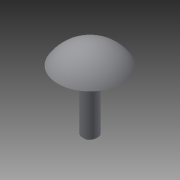
# Autodesk Inventor part: Linkage Peg
Saved by Autodesk Inventor 2015 (Build 190159000, 159)
## iProperties
Created: 2018-03-27
Part Number: Linkage Peg
Material: Generic
Document SubType Name: Modeling
Designer: Administrator
Density: 1 g/cm^3
Appearance: Default
Author: Administrator
Autodesk Inventor part; units mm, degrees
ref_plane "YZ Plane" through (0, 0, 0) normal (1, 0, 0) x (0, 1, 0)
ref_plane "XZ Plane" through (0, 0, 0) normal (0, 1, 0) x (-1, 0, 0)
ref_plane "XY Plane" through (0, 0, 0) normal (0, 0, 1) x (1, 0, 0)
sketch "Sketch1" plane through (0, 0, 0) normal (0, 0, 1) x (1, 0, 0)
  line L0 (0, 0) -> (0, 8.255)
  line L1 (0, 0) -> (0.7938, 0)
  line L2 (0.7938, 0) -> (0.7937, 6.35)
  arc A0 (3.3337, 6.35) -> (0, 8.255) centre (-0.0557, 4.2879) ccw
  line L3 (0.7937, 6.35) -> (3.3337, 6.35)
  dimension "d0" = 3.9675
  dimension "d1" = 6.35
  dimension "d2" = 8.255
  dimension "d3" = 0.7937
  dimension "d4" = 2.54
  constraints: 8 end point, 2 horizontal, 2 point on circle, 1 centre point, 1 perpendicular, 1 vertical
  measures "d0" radius of A0
  measures "d1" distance of L1.end L2.end
  measures "d2" distance of L0.start L0.end
  measures "d3" distance between parallel lines of L2 L0
  measures "d4" distance of L2.end L3.end
revolve "Revolution1" add sketch "Sketch1" angle 360 about axis through (0, 0, 0) along (0, 1, 0)
chamfer "Chamfer1" distance 0.254 angle 45 1 edges at (-0.7938, 0, 0)
body "Solid1"
